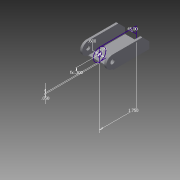
# Autodesk Inventor part: LegHolderV2
Saved by Autodesk Inventor 2014 (Build 180170000, 170)
## iProperties
Created: 2014-04-24
Part Number: LegHolderV2
Material: Generic
Document SubType Name: Modeling
Designer: Max
Density: 1 g/cm^3
Appearance: Default
Author: Max
Autodesk Inventor part; units mm, degrees
ref_plane "YZ Plane" through (0, 0, 0) normal (1, 0, 0) x (0, 1, 0)
ref_plane "XZ Plane" through (0, 0, 0) normal (0, 1, 0) x (-1, 0, 0)
ref_plane "XY Plane" through (0, 0, 0) normal (0, 0, 1) x (1, 0, 0)
sketch "Sketch1" plane through (0, 0, 0) normal (1, 0, 0) x (0, 1, 0)
  line L0 (0, 0) -> (16.51, 0)
  line L1 (16.51, 0) -> (16.51, 44.45)
  line L2 (16.51, 44.45) -> (0, 44.45)
  line L3 (0, 44.45) -> (0, 0)
  line L4 (1.27, 44.45) -> (1.27, 0)
  circle A0 centre (8.89, 44.45) radius 7.62
  line L5 (0, 44.45) -> (2.3586, 48.3749)
  circle A1 centre (8.89, 44.45) radius 2.54
  line L6 (8.255, 0) -> (16.51, 8.255)
  dimension "d2" = 15.24
  dimension "d0" = 44.45
  dimension "d1" = 1.27
  dimension "d3" = 7.62
  dimension "d4" = 5.08
  dimension "d5" = 45
  constraints: 14 end point, 4 point on line, 2 parallel, 2 perpendicular, 1 centre point, 1 coincident, 1 horizontal, 1 midpoint, 1 vertical, 4 other
  measures "d0" distance between parallel lines of L0 L2
  measures "d1" distance between parallel lines of L3 L4
  measures "d3" distance from line of L4 point (8.89, 44.45)
  measures "d4" diameter of A1
  measures "d5" angle of L1 L6
extrude "Extrusion1" add sketch "Sketch1" along normal mid plane 31.75 contours L3 L2 L4 L0 | L4 A0 L1 L6 L0 | A0 L2 A1 | L2 A1 A0 | A1 L2 | L2 A1
extrude "Extrusion2" cut sketch "Sketch1" along normal through all both and the other way through all contours A1 L2 | L2 A1
extrude "Extrusion3" cut sketch "Sketch1" along normal mid plane 26.67 contours L4 A0 L1 L6 L0 | A0 L2 A1 | L2 A1 A0 | L2 A1 picked at (9.5237, 43.4833)
equation "\"d3\" = 0.5 * d2"
body "Solid1"
